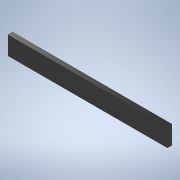
# Autodesk Inventor part: рот
Saved by Autodesk Inventor 2021.1 (Build 251245010, 245A)
## iProperties
Created: 2023-01-21
Part Number: рот
Material: Типовые
Document SubType Name: Modeling
Designer: zmoze
Density: 1 g/cm^3
Appearance: Глянцевая - черная
Author: zmoze
Autodesk Inventor part; units mm, degrees
ref_plane "YZ Plane" through (0, 0, 0) normal (1, 0, 0) x (0, 1, 0)
ref_plane "XZ Plane" through (0, 0, 0) normal (0, 1, 0) x (-1, 0, 0)
ref_plane "XY Plane" through (0, 0, 0) normal (0, 0, 1) x (1, 0, 0)
sketch "Эскиз1" plane through (0, 0, 0) normal (0, 0, 1) x (1, 0, 0)
  line L0 (-52.25, 6) -> (52.25, 6)
  line L1 (52.25, 6) -> (52.25, -6)
  line L2 (52.25, -6) -> (-52.25, -6)
  line L3 (-52.25, -6) -> (-52.25, 6)
  line L4 (-52.25, 6) -> (52.25, -6) construction
  line L5 (52.25, 6) -> (-52.25, -6) construction
  point P0 (0, 0)
  dimension "d0" = 104.5
  dimension "d1" = 12
  constraints: 12 end point, 2 midpoint, 2 parallel, 1 horizontal, 1 perpendicular
  measures "d0" distance of L0.start L0.end
  measures "d1" distance of L2.end L0.start
extrude "Выдавливание1" add sketch "Эскиз1" along normal blind 3
